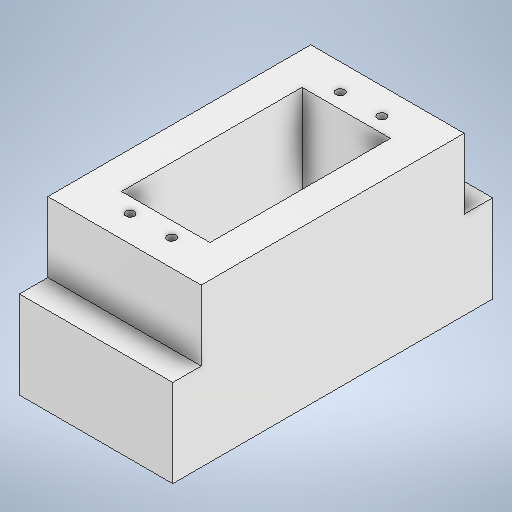
# Autodesk Inventor part: Base_servo_efector
Saved by Autodesk Inventor 2025.1 (Build 291241000, 241)
## iProperties
Created: 2024-12-10
Part Number: Base_servo_efector
Material: Acetal Resin, White
Document SubType Name: Modeling
Designer: Cristhian Vigo
Density: 1.425 g/cm^3
Appearance: Smooth - White
Author: Cristhian Vigo
Autodesk Inventor part; units mm, degrees
ref_plane "YZ Plane" through (0, 0, 0) normal (1, 0, 0) x (0, 1, 0)
ref_plane "XZ Plane" through (0, 0, 0) normal (0, 1, 0) x (-1, 0, 0)
ref_plane "XY Plane" through (0, 0, 0) normal (0, 0, 1) x (1, 0, 0)
sketch "Sketch1" plane through (0, 0, 0) normal (0, 1, 0) x (-1, 0, 0)
  line L0 (-17.5, -36.5) -> (17.5, -36.5)
  line L1 (17.5, -36.5) -> (17.5, 36.5)
  line L2 (17.5, 36.5) -> (-17.5, 36.5)
  line L3 (-17.5, 36.5) -> (-17.5, -36.5)
  line L4 (-17.5, -36.5) -> (17.5, 36.5) construction
  line L5 (17.5, -36.5) -> (-17.5, 36.5) construction
  point P0 (0, 0)
  dimension "d0" = 35
  dimension "d1" = 73
  constraints: 12 end point, 2 midpoint, 2 parallel, 1 horizontal, 1 perpendicular
  measures "d0" distance of L2.end L1.end
  measures "d1" distance of L1.end L0.end
extrude "Extrusion1" add sketch "Sketch1" along normal blind 6
sketch "Sketch2" plane through (0, 6, 0) normal (0, 1, 0) x (1, 0, 0)
  line L0 (14.5, 25) -> (-14.5, 25)
  line L1 (-14.5, 25) -> (-14.5, -25)
  line L2 (-14.5, -25) -> (14.5, -25)
  line L3 (14.5, -25) -> (14.5, 25)
  line L4 (14.5, 25) -> (-14.5, -25) construction
  line L5 (-14.5, 25) -> (14.5, -25) construction
  line L6 (-17.5, 36.5) -> (-17.5, -36.5) projected
  line L7 (17.5, -36.5) -> (17.5, 36.5) projected
  line L8 (-17.5, -36.5) -> (17.5, -36.5)
  line L9 (17.5, -36.5) -> (17.5, -30.5)
  line L10 (17.5, -30.5) -> (-17.5, -30.5)
  line L11 (-17.5, -30.5) -> (-17.5, -36.5)
  line L12 (-17.5, 36.5) -> (17.5, 36.5)
  line L13 (17.5, 36.5) -> (17.5, 30.5)
  line L14 (17.5, 30.5) -> (-17.5, 30.5)
  line L15 (-17.5, 30.5) -> (-17.5, 36.5)
  point P0 (0, 0)
  dimension "d4" = 29
  dimension "d5" = 50
  dimension "d15" = 6
  dimension "d16" = 6
  constraints: 28 end point, 6 parallel, 3 horizontal, 3 perpendicular, 3 point on line, 2 midpoint
  measures "d4" distance of L2.end L1.end
  measures "d5" distance of L1.end L0.end
  measures "d15" distance of L9.end L8.end
  measures "d16" distance of L12.end L13.end
extrude "Extrusion2" add sketch "Sketch2" along normal blind 14
sketch "Sketch4" plane through (0, 6, 0) normal (0, 1, 0) x (1, 0, 0)
  circle A0 centre (0, 0) radius 6
  line L0 (15, 24.0075) -> (-15, 24.0075)
  line L1 (-15, 24.0075) -> (-15, -24.0075)
  line L2 (-15, -24.0075) -> (15, -24.0075)
  line L3 (15, -24.0075) -> (15, 24.0075)
  line L4 (15, 24.0075) -> (-15, -24.0075) construction
  line L5 (-15, 24.0075) -> (15, -24.0075) construction
  circle A1 centre (-10, -18.6005) radius 1.4
  line L6 (-14.5, -25) -> (-14.5, 25) projected
  circle A2 centre (-8, -8.5005) radius 1.4
  line L7 (12.9011, 0) -> (-11.0407, 0) construction
  line L8 (0, -11.5905) -> (0, 16.5955) construction
  circle A3 centre (-10, 18.6005) radius 1.4
  circle A4 centre (-8, 8.5005) radius 1.4
  circle A5 centre (10, -18.6005) radius 1.4
  circle A6 centre (8, -8.5005) radius 1.4
  circle A7 centre (10, 18.6005) radius 1.4
  circle A8 centre (8, 8.5005) radius 1.4
  dimension "d19" = 12
  dimension "d20" = 30
  dimension "d21" = 48.015
  dimension "d22" = 2.8
  dimension "d23" = 4.5
  dimension "d24" = 4.007
  dimension "d25" = 2.8
  dimension "d26" = 6.5
  dimension "d27" = 15.507
  constraints: 16 end point, 9 centre point, 6 symmetric about line, 2 horizontal, 2 midpoint, 2 parallel, 1 perpendicular, 1 vertical, 7 other
  measures "d19" diameter of A0
  measures "d20" distance of L2.end L1.end
  measures "d21" distance of L1.end L0.end
  measures "d22" diameter of A1
  measures "d23" distance from line of L6 A1.centre
  measures "d24" distance edge to line of A1 L2
  measures "d25" diameter of A2
  measures "d26" distance from line of L6 A2.centre
  measures "d27" distance from line of L2 A2.centre
extrude "Extrusion4" cut sketch "Sketch4" against normal through all contours A0 | A1 | A2 | A3 | A4 | A5 | A6 | A7 | A8
sketch "Sketch9" plane through (0, 20, 0) normal (0, 1, 0) x (1, 0, 0)
  line L0 (-14.5, -25) -> (-14.5, 25) projected
  line L1 (14.5, -25) -> (-14.5, -25)
  line L2 (-14.5, -25) -> (-14.5, 25)
  line L3 (-14.5, 25) -> (14.5, 25)
  line L4 (14.5, 25) -> (14.5, -25)
  line L5 (14.5, -25) -> (-14.5, 25) construction
  line L6 (-14.5, -25) -> (14.5, 25) construction
  line L7 (10.1, -20.6) -> (-10.1, -20.6)
  line L8 (-10.1, -20.6) -> (-10.1, 20.6)
  line L9 (-10.1, 20.6) -> (10.1, 20.6)
  line L10 (10.1, 20.6) -> (10.1, -20.6)
  line L11 (10.1, -20.6) -> (-10.1, 20.6) construction
  line L12 (-10.1, -20.6) -> (10.1, 20.6) construction
  point P0 (0, 0)
  dimension "d45" = 20.2
  dimension "d46" = 41.2
  constraints: 24 end point, 4 midpoint, 4 parallel, 2 horizontal, 2 perpendicular
  measures "d45" distance of L8.end L9.end
  measures "d46" distance of L7.end L8.end
extrude "Extrusion8" add sketch "Sketch9" along normal blind 16 and the other way blind 10
sketch "Sketch10" plane through (0, 20, 0) normal (0, 1, 0) x (1, 0, 0)
  line L0 (-14.5, 25) -> (14.5, 25) projected
  line L1 (14.5, -25) -> (-14.5, -25)
  line L2 (-14.5, -25) -> (-14.5, 25)
  line L3 (-14.5, 25) -> (14.5, 25)
  line L4 (14.5, 25) -> (14.5, -25)
  line L5 (14.5, -25) -> (-14.5, 25) construction
  line L6 (-14.5, -25) -> (14.5, 25) construction
  line L7 (17.5, -30) -> (-17.5, -30)
  line L8 (-17.5, -30) -> (-17.5, 30)
  line L9 (-17.5, 30) -> (17.5, 30)
  line L10 (17.5, 30) -> (17.5, -30)
  line L11 (17.5, -30) -> (-17.5, 30) construction
  line L12 (-17.5, -30) -> (17.5, 30) construction
  point P0 (0, 0)
  point P1 (14.5, 25)
  dimension "d51" = 35
  dimension "d52" = 60
  constraints: 24 end point, 4 midpoint, 4 parallel, 2 horizontal, 2 perpendicular
  measures "d51" distance of L8.end L9.end
  measures "d52" distance of L7.end L8.end
extrude "Extrusion9" add sketch "Sketch10" along normal up to surface (16 mm away)
sketch "Sketch12" plane through (0, 36, 0) normal (0, 1, 0) x (1, 0, 0)
  line L0 (4.75, -24) -> (-4.75, -24)
  line L1 (-4.75, -24) -> (-4.75, 24)
  line L2 (-4.75, 24) -> (4.75, 24)
  line L3 (4.75, 24) -> (4.75, -24)
  line L4 (4.75, -24) -> (-4.75, 24) construction
  line L5 (-4.75, -24) -> (4.75, 24) construction
  point P0 (0, 0)
  dimension "d55" = 9.5
  dimension "d56" = 48
  constraints: 12 end point, 4 coincident, 2 midpoint, 2 parallel, 1 horizontal, 1 perpendicular
  measures "d55" distance of L1.end L2.end
  measures "d56" distance of L0.end L1.end
hole "Hole1" at (-4.75, 36, -24) at (4.75, 36, -24) at (-4.75, 36, 24) at (4.75, 36, 24) direction (0, -1, 0) diameter 2 depth 15
equation "\"d1\" = Esla_Bas_Largo"
equation "\"Esla_Bas_Largo\" = 73"
body "Solid1"
